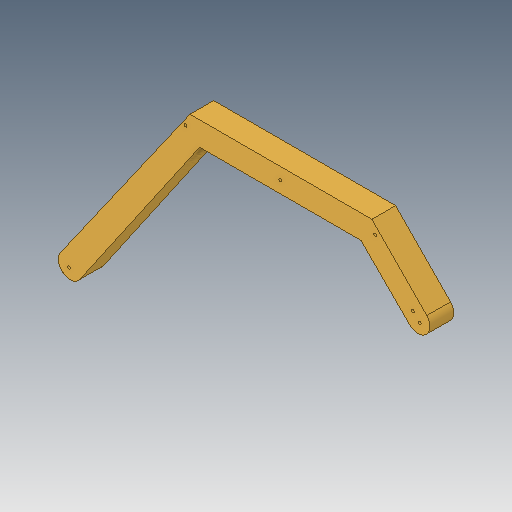
# Autodesk Inventor part: bodi metal
Saved by Autodesk Inventor 2018 (Build 220112000, 112)
## iProperties
Created: 2019-12-19
Part Number: bodi metal
Material: Generic
Document SubType Name: Modeling
Designer: Ibnu
Density: 1 g/cm^3
Appearance: Default
Mass: 310.493 g
Surface Area: 526.556 cm^2
Volume: 310.493 cm^3
Author: Ibnu
Autodesk Inventor part; units mm, degrees
ref_plane "YZ Plane" through (0, 0, 0) normal (1, 0, 0) x (0, 1, 0)
ref_plane "XZ Plane" through (0, 0, 0) normal (0, 1, 0) x (-1, 0, 0)
ref_plane "XY Plane" through (0, 0, 0) normal (0, 0, 1) x (1, 0, 0)
sketch "Sketch1" plane through (0, 0, 0) normal (0, 0, 1) x (1, 0, 0)
  line L0 (176.7767, 176.7767) -> (346.7767, 176.7767)
  line L1 (346.7767, 176.7767) -> (406.8808, 116.6726)
  line L2 (176.7767, 201.7767) -> (346.7767, 201.7767)
  line L3 (406.8808, 116.6726) -> (424.5584, 134.3503)
  line L4 (424.5584, 134.3503) -> (358.3302, 201.7767)
  line L5 (358.3302, 201.7767) -> (346.7767, 201.7767)
  line L6 (166.5538, 201.7767) -> (176.7767, 201.7767)
  circle A0 centre (408.6485, 132.5825) radius 1.5
  circle A1 centre (401.5775, 139.6536) radius 1.5
  line L7 (166.5538, 201.7767) -> (22.9408, -2.8578)
  line L8 (22.9408, -2.8578) -> (43.4042, -17.2191)
  line L9 (43.4042, -17.2191) -> (176.7767, 176.7767)
  circle A2 centre (38.917, -1.8531) radius 1.5
  circle A3 centre (161.7767, 189.2767) radius 1.5
  circle A4 centre (361.7767, 189.2767) radius 1.5
  circle A5 centre (261.7767, 189.2767) radius 1.5
  dimension "d32" = 3
  dimension "d33" = 3
  dimension "d37" = 3
  constraints: 20 end point, 6 centre point, 2 collinear, 1 horizontal, 1 perpendicular, 1 point on line
  measures "d32" diameter of A3
  measures "d33" diameter of A4
  measures "d37" diameter of A5
extrude "Extrusion5" add sketch "Sketch1" along normal blind 25
fillet "Fillet6" radius 12 4 edges at (22.9408, -2.8578, 12.5) (43.4042, -17.2191, 12.5) (406.8808, 116.6726, 12.5) (424.5584, 134.3503, 12.5)
body "Solid4"
